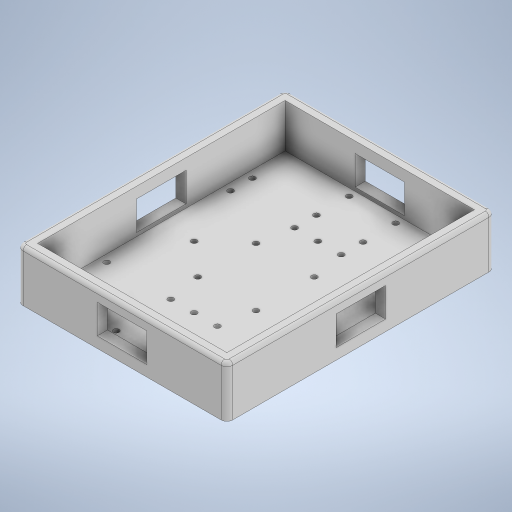
# Autodesk Inventor part: base
Saved by Autodesk Inventor 2024 (Build 280153000, 153)
## iProperties
Created: 2023-11-06
Part Number: base
Material: Generic
Document SubType Name: Modeling
Designer: dimademler
Density: 1 g/cm^3
Appearance: Default
Author: dimademler
Autodesk Inventor part; units mm, degrees
ref_plane "YZ Plane" through (0, 0, 0) normal (1, 0, 0) x (0, 1, 0)
ref_plane "XZ Plane" through (0, 0, 0) normal (0, 1, 0) x (-1, 0, 0)
ref_plane "XY Plane" through (0, 0, 0) normal (0, 0, 1) x (1, 0, 0)
sketch "Sketch2" plane through (0, 0, 0) normal (0, 1, 0) x (-1, 0, 0)
  line L0 (0, 0) -> (177.8, 0)
  line L1 (177.8, 0) -> (177.8, 228.6)
  line L2 (177.8, 228.6) -> (0, 228.6)
  line L3 (0, 228.6) -> (0, 0)
  dimension "d0" = 177.8
  dimension "d1" = 228.6
  constraints: 8 end point, 2 parallel, 1 horizontal, 1 perpendicular
  measures "d0" distance of L2.end L1.end
  measures "d1" distance of L1.end L0.end
extrude "Extrusion1" add sketch "Sketch2" along normal blind 6.35
sketch "Sketch3" plane through (0, 6.35, 0) normal (0, 1, 0) x (1, 0, 0)
  line L0 (-177.8, -228.6) -> (0, -228.6) projected
  line L1 (-177.8, 0) -> (-177.8, -228.6) projected
  line L2 (0, 0) -> (-177.8, 0) projected
  line L3 (0, -228.6) -> (0, 0) projected
  line L4 (-88.9, -228.6) -> (-88.9, -222.25) construction
  line L5 (-88.9, 0) -> (-88.9, -6.35) construction
  line L6 (-177.8, -114.3) -> (-171.45, -114.3) construction
  line L7 (0, -114.3) -> (-6.35, -114.3) construction
  line L8 (-171.45, -114.3) -> (-171.45, -6.35)
  line L9 (-171.45, -114.3) -> (-171.45, -222.25)
  line L10 (-171.45, -6.35) -> (-88.9, -6.35)
  line L11 (-6.35, -6.35) -> (-88.9, -6.35)
  line L12 (-6.35, -6.35) -> (-6.35, -114.3)
  line L13 (-6.35, -114.3) -> (-6.35, -222.25)
  line L14 (-6.35, -222.25) -> (-88.9, -222.25)
  line L15 (-171.45, -222.25) -> (-88.9, -222.25)
  line L16 (-177.8, -228.6) -> (0, -228.6)
  line L17 (0, -228.6) -> (0, 0)
  line L18 (0, 0) -> (-177.8, 0)
  line L19 (-177.8, 0) -> (-177.8, -228.6)
  dimension "d4" = 6.35
  dimension "d5" = 6.35
  dimension "d6" = 6.35
  dimension "d7" = 6.35
  constraints: 32 end point, 5 vertical, 4 equal length, 4 horizontal, 4 midpoint, 2 perpendicular, 2 point on line
  measures "d4" distance of L4.start L4.end
  measures "d5" distance of L5.start L5.end
  measures "d6" distance of L6.start L6.end
  measures "d7" distance of L7.start L7.end
extrude "Extrusion2" add sketch "Sketch3" along normal blind 38.1
sketch "Sketch4" plane through (0, 0, 0) normal (0, -1, 0) x (1, 0, 0)
  line L0 (-177.8, 0) -> (-177.8, 228.6) projected
  line L1 (-177.8, 228.6) -> (0, 228.6) construction
  line L2 (0, 228.6) -> (0, 0) projected
  line L3 (0, 0) -> (-177.8, 0) projected
  line L4 (-88.9, 228.6) -> (-88.9, 0) construction
  line L5 (0, 114.3) -> (-177.8, 114.3) construction
  line L6 (-88.9, 228.6) -> (-68.58, 228.6)
  line L7 (0, 228.6) -> (-177.8, 228.6) construction
  line L8 (-88.9, 228.6) -> (-109.22, 228.6)
  line L9 (-68.58, 228.6) -> (-68.58, 0) construction
  line L10 (-109.22, 228.6) -> (-109.22, 0) construction
  line L11 (-68.58, 228.6) -> (-68.58, 177.8) construction
  line L12 (-109.22, 228.6) -> (-109.22, 177.8) construction
  line L13 (-68.58, 177.8) -> (-68.58, 187.325) construction
  line L14 (-68.58, 177.8) -> (-68.58, 168.275) construction
  circle A0 centre (-68.58, 187.325) radius 2.413
  circle A1 centre (-68.58, 168.275) radius 2.413
  line L15 (-68.58, 187.325) -> (0, 187.325) construction
  line L16 (0, 187.325) -> (-12.7, 187.325) construction
  line L17 (-68.58, 168.275) -> (0, 168.275) construction
  line L18 (0, 168.275) -> (-12.7, 168.275) construction
  circle A2 centre (-12.7, 187.325) radius 2.413
  circle A3 centre (-12.7, 168.275) radius 2.413
  circle A4 centre (-68.58, 215.9) radius 2.413
  circle A5 centre (-109.22, 187.325) radius 2.413
  circle A6 centre (-109.22, 168.275) radius 2.413
  circle A7 centre (-165.1, 187.325) radius 2.413
  circle A8 centre (-165.1, 168.275) radius 2.413
  circle A9 centre (-109.22, 215.9) radius 2.413
  circle A10 centre (-68.58, 41.275) radius 2.413
  circle A11 centre (-68.58, 60.325) radius 2.413
  circle A12 centre (-12.7, 41.275) radius 2.413
  circle A13 centre (-12.7, 60.325) radius 2.413
  circle A14 centre (-68.58, 12.7) radius 2.413
  circle A15 centre (-109.22, 12.7) radius 2.413
  circle A16 centre (-109.22, 41.275) radius 2.413
  circle A17 centre (-165.1, 41.275) radius 2.413
  circle A18 centre (-165.1, 60.325) radius 2.413
  circle A19 centre (-109.22, 60.325) radius 2.413
  dimension "d10" = 20.32
  dimension "d11" = 50.8
  dimension "d12" = 9.525
  dimension "d13" = 4.826
  dimension "d14" = 4.826
  dimension "d16" = 12.7
  dimension "d17" = 4.826
  dimension "d18" = 4.826
  dimension "d19" = 12.7
  dimension "d20" = 4.826
  dimension "d21" = 12.7
  constraints: 30 end point, 20 centre point, 19 symmetric about line, 12 point on line, 4 coincident, 4 midpoint, 2 equal length, 2 perpendicular, 1 parallel, 15 other
  measures "d10" distance of L4.start L6.end
  measures "d11" distance of L6.end L11.end
  measures "d12" distance of L11.end L13.end
  measures "d13" diameter of A0
  measures "d14" diameter of A1
  measures "d16" distance of L15.end L16.end
  measures "d17" diameter of A2
  measures "d18" diameter of A3
  measures "d19" distance of L17.end L18.end
  measures "d20" diameter of A4
  measures "d21" distance from line of L6 A4.centre
extrude "Extrusion3" cut sketch "Sketch4" against normal through all
sketch "Sketch5" plane through (0, 6.35, 0) normal (0, 1, 0) x (1, 0, 0)
  circle A0 centre (-109.22, -187.325) radius 2.413 projected
  circle A1 centre (-68.58, -168.275) radius 2.413 projected
  circle A2 centre (-12.7, -60.325) radius 2.413 projected
  circle A3 centre (-68.58, -12.7) radius 2.413 projected
  circle A4 centre (-165.1, -60.325) radius 2.413 projected
  circle A5 centre (-109.22, -60.325) radius 2.413 projected
  circle A6 centre (-68.58, -60.325) radius 2.413 projected
  circle A7 centre (-12.7, -168.275) radius 2.413 projected
  circle A8 centre (-109.22, -168.275) radius 2.413 projected
  circle A9 centre (-109.22, -215.9) radius 2.413 projected
  circle A10 centre (-165.1, -187.325) radius 2.413 projected
  circle A11 centre (-68.58, -187.325) radius 2.413 projected
  circle A12 centre (-12.7, -41.275) radius 2.413 projected
  circle A13 centre (-109.22, -12.7) radius 2.413 projected
  circle A14 centre (-165.1, -41.275) radius 2.413 projected
  circle A15 centre (-109.22, -41.275) radius 2.413 projected
  circle A16 centre (-68.58, -41.275) radius 2.413 projected
  circle A17 centre (-12.7, -187.325) radius 2.413 projected
  circle A18 centre (-165.1, -168.275) radius 2.413 projected
  circle A19 centre (-68.58, -215.9) radius 2.413 projected
  line L0 (-171.45, -222.25) -> (-6.35, -222.25) projected
  line L1 (-6.35, -222.25) -> (-6.35, -6.35) projected
  line L2 (-6.35, -6.35) -> (-171.45, -6.35) projected
  line L3 (-171.45, -6.35) -> (-171.45, -222.25) projected
  line L4 (-171.45, -114.3) -> (-6.35, -114.3) construction
  line L5 (-88.9, -6.35) -> (-88.9, -222.25) construction
  line L6 (-34.925, -168.275) -> (-142.875, -168.275) construction
  line L7 (-142.875, -168.275) -> (-142.875, -60.325) construction
  line L8 (-142.875, -60.325) -> (-34.925, -60.325) construction
  line L9 (-34.925, -60.325) -> (-34.925, -168.275) construction
  line L10 (-34.925, -168.275) -> (-142.875, -60.325) construction
  line L11 (-142.875, -168.275) -> (-34.925, -60.325) construction
  circle A20 centre (-88.9, -168.275) radius 2.413
  circle A21 centre (-142.875, -114.3) radius 2.413
  circle A22 centre (-88.9, -60.325) radius 2.413
  circle A23 centre (-34.925, -114.3) radius 2.413
  point P0 (0, 0)
  point P1 (-88.9, -114.3)
  dimension "d24" = 107.95
  dimension "d25" = 107.95
  dimension "d26" = 4.826
  dimension "d27" = 4.826
  dimension "d28" = 4.826
  dimension "d29" = 4.826
  constraints: 16 end point, 11 midpoint, 4 centre point, 2 parallel, 1 horizontal, 1 perpendicular
  measures "d24" distance of L7.end L8.end
  measures "d25" distance of L6.end L7.end
  measures "d26" diameter of A20
  measures "d27" diameter of A21
  measures "d28" diameter of A22
  measures "d29" diameter of A23
extrude "Extrusion4" cut sketch "Sketch5" against normal blind 6.35 contours A20 | A21 | A22 | A23
sketch "Sketch8" plane through (0, 6.35, 0) normal (0, 1, 0) x (1, 0, 0)
  circle A0 centre (-88.9, -168.275) radius 2.413 projected
  circle A1 centre (-88.9, -60.325) radius 2.413 projected
  circle A2 centre (-34.925, -114.3) radius 2.413 projected
  circle A3 centre (-142.875, -114.3) radius 2.413 projected
  circle A4 centre (-109.22, -187.325) radius 2.413 projected
  circle A5 centre (-68.58, -168.275) radius 2.413 projected
  circle A6 centre (-12.7, -60.325) radius 2.413 projected
  circle A7 centre (-68.58, -12.7) radius 2.413 projected
  circle A8 centre (-165.1, -60.325) radius 2.413 projected
  circle A9 centre (-109.22, -60.325) radius 2.413 projected
  circle A10 centre (-68.58, -60.325) radius 2.413 projected
  circle A11 centre (-12.7, -168.275) radius 2.413 projected
  circle A12 centre (-109.22, -168.275) radius 2.413 projected
  circle A13 centre (-109.22, -215.9) radius 2.413 projected
  circle A14 centre (-165.1, -187.325) radius 2.413 projected
  circle A15 centre (-68.58, -187.325) radius 2.413 projected
  circle A16 centre (-12.7, -41.275) radius 2.413 projected
  circle A17 centre (-109.22, -12.7) radius 2.413 projected
  circle A18 centre (-165.1, -41.275) radius 2.413 projected
  circle A19 centre (-109.22, -41.275) radius 2.413 projected
  circle A20 centre (-68.58, -41.275) radius 2.413 projected
  circle A21 centre (-12.7, -187.325) radius 2.413 projected
  circle A22 centre (-165.1, -168.275) radius 2.413 projected
  circle A23 centre (-68.58, -215.9) radius 2.413 projected
  line L0 (-171.45, -222.25) -> (-6.35, -222.25) projected
  line L1 (-6.35, -222.25) -> (-6.35, -6.35) projected
  line L2 (-6.35, -6.35) -> (-171.45, -6.35) projected
  line L3 (-171.45, -6.35) -> (-171.45, -222.25) projected
  line L4 (-142.875, -114.3) -> (-34.925, -114.3) construction
  line L5 (-88.9, -60.325) -> (-88.9, -168.275) construction
  line L6 (-114.3, -88.9) -> (-63.5, -88.9) construction
  line L7 (-63.5, -88.9) -> (-63.5, -139.7) construction
  line L8 (-63.5, -139.7) -> (-114.3, -139.7) construction
  line L9 (-114.3, -139.7) -> (-114.3, -88.9) construction
  line L10 (-114.3, -88.9) -> (-63.5, -139.7) construction
  line L11 (-63.5, -88.9) -> (-114.3, -139.7) construction
  circle A24 centre (-114.3, -88.9) radius 2.413
  circle A25 centre (-63.5, -88.9) radius 2.413
  circle A26 centre (-114.3, -139.7) radius 2.413
  circle A27 centre (-63.5, -139.7) radius 2.413
  point P0 (0, 0)
  point P1 (-88.9, -114.3)
  dimension "d38" = 50.8
  dimension "d39" = 50.8
  dimension "d40" = 4.826
  dimension "d41" = 4.826
  dimension "d42" = 4.826
  dimension "d43" = 4.826
  constraints: 16 end point, 4 centre point, 4 coincident, 3 midpoint, 2 horizontal, 2 parallel, 1 perpendicular, 1 vertical
  measures "d38" distance of L7.end L8.end
  measures "d39" distance of L6.end L7.end
  measures "d40" diameter of A24
  measures "d41" diameter of A25
  measures "d42" diameter of A26
  measures "d43" diameter of A27
extrude "Extrusion7" cut sketch "Sketch8" against normal through all contours A24 | A25 | A26 | A27
sketch "Sketch9" plane through (-177.8, 0, 228.6) normal (0, 0, 1) x (1, 0, 0)
  line L0 (177.8, 44.45) -> (0, 44.45) projected
  line L1 (88.9, 44.45) -> (88.9, 0) construction
  line L2 (91.313, 0) -> (86.487, 0) projected
  line L3 (177.8, 0) -> (177.8, 44.45) projected
  line L4 (0, 0) -> (0, 44.45) projected
  line L5 (177.8, 22.225) -> (0, 22.225) construction
  line L6 (67.31, 9.525) -> (110.49, 9.525)
  line L7 (110.49, 9.525) -> (110.49, 34.925)
  line L8 (110.49, 34.925) -> (67.31, 34.925)
  line L9 (67.31, 34.925) -> (67.31, 9.525)
  line L10 (67.31, 9.525) -> (110.49, 34.925) construction
  line L11 (110.49, 9.525) -> (67.31, 34.925) construction
  point P0 (88.9, 22.225)
  dimension "d46" = 43.18
  dimension "d47" = 25.4
  constraints: 16 end point, 7 midpoint, 2 parallel, 1 horizontal, 1 perpendicular
  measures "d46" distance of L7.end L8.end
  measures "d47" distance of L6.end L7.end
extrude "Extrusion8" cut sketch "Sketch9" against normal through all
sketch "Sketch10" plane through (0, 0, 228.6) normal (1, 0, 0) x (0, 0, -1)
  line L0 (0, 0) -> (228.6, 0) projected
  line L1 (228.6, 0) -> (228.6, 44.45) projected
  line L2 (0, 44.45) -> (228.6, 44.45) projected
  line L3 (0, 0) -> (0, 44.45) projected
  line L4 (0, 22.225) -> (228.6, 22.225) construction
  line L5 (114.3, 44.45) -> (114.3, 0) construction
  line L6 (92.71, 9.525) -> (135.89, 9.525)
  line L7 (135.89, 9.525) -> (135.89, 34.925)
  line L8 (135.89, 34.925) -> (92.71, 34.925)
  line L9 (92.71, 34.925) -> (92.71, 9.525)
  line L10 (92.71, 9.525) -> (135.89, 34.925) construction
  line L11 (135.89, 9.525) -> (92.71, 34.925) construction
  point P0 (114.3, 22.225)
  dimension "d50" = 43.18
  dimension "d51" = 25.4
  constraints: 16 end point, 7 midpoint, 2 parallel, 1 horizontal, 1 perpendicular
  measures "d50" distance of L8.end L7.end
  measures "d51" distance of L7.end L6.end
extrude "Extrusion9" cut sketch "Sketch10" against normal through all contours L9 L8 L7 L6
sketch "Sketch11" plane through (-177.8, 0, 228.6) normal (0, 0, 1) x (1, 0, 0)
  line L0 (67.31, 34.925) -> (110.49, 34.925) projected
  line L1 (110.49, 34.925) -> (110.49, 9.525) projected
  line L2 (110.49, 9.525) -> (67.31, 9.525) projected
  line L3 (67.31, 9.525) -> (67.31, 34.925) projected
  line L4 (0, 0) -> (177.8, 0) projected
  line L5 (177.8, 0) -> (177.8, 44.45) projected
  line L6 (0, 44.45) -> (177.8, 44.45) projected
  line L7 (0, 0) -> (0, 44.45) projected
  point P0 (177.8, 0)
extrude "Extrusion10" add sketch "Sketch11" along normal blind 2.54
sketch "Sketch12" plane through (0, 0, 0) normal (1, 0, 0) x (0, 0, -1)
  line L0 (-135.89, 34.925) -> (-92.71, 34.925) projected
  line L1 (-92.71, 34.925) -> (-92.71, 9.525) projected
  line L2 (-92.71, 9.525) -> (-135.89, 9.525) projected
  line L3 (-135.89, 9.525) -> (-135.89, 34.925) projected
  line L4 (0, 0) -> (-231.14, 0) projected
  line L5 (0, 0) -> (0, 44.45) projected
  line L6 (0, 44.45) -> (-231.14, 44.45) projected
  line L7 (-231.14, 0) -> (-231.14, 44.45) projected
  line L8 (0, 34.925) -> (0, 9.525) projected
  line L9 (0, 9.525) -> (0, 34.925) projected
  line L10 (0, 0) -> (0, 44.45) projected
  line L11 (0, 0) -> (0, 44.45) projected
extrude "Extrusion11" add sketch "Sketch12" along normal blind 2.54
sketch "Sketch13" plane through (-177.8, 0, 0) normal (0, 0, -1) x (-1, 0, 0)
  line L0 (-110.49, 34.925) -> (-67.31, 34.925) projected
  line L1 (-67.31, 34.925) -> (-67.31, 9.525) projected
  line L2 (-67.31, 9.525) -> (-110.49, 9.525) projected
  line L3 (-110.49, 9.525) -> (-110.49, 34.925) projected
  line L4 (0, 0) -> (-180.34, 0) projected
  line L5 (0, 0) -> (0, 44.45) projected
  line L6 (0, 44.45) -> (-180.34, 44.45) projected
  line L7 (-180.34, 0) -> (-180.34, 44.45) projected
  point P0 (-177.8, 0)
extrude "Extrusion12" add sketch "Sketch13" along normal blind 2.54
sketch "Sketch14" plane through (-177.8, 0, 231.14) normal (-1, 0, 0) x (0, 0, 1)
  line L0 (-138.43, 34.925) -> (-95.25, 34.925) projected
  line L1 (-95.25, 34.925) -> (-95.25, 9.525) projected
  line L2 (-95.25, 9.525) -> (-138.43, 9.525) projected
  line L3 (-138.43, 9.525) -> (-138.43, 34.925) projected
  line L4 (-233.68, 0) -> (0, 0) projected
  line L5 (0, 44.45) -> (0, 0) projected
  line L6 (0, 44.45) -> (-233.68, 44.45) projected
  line L7 (-233.68, 0) -> (-233.68, 44.45) projected
  point P0 (-231.14, 0)
extrude "Extrusion13" add sketch "Sketch14" along normal blind 2.54
fillet "Fillet1" radius 5.08 1 edges at (-180.34, 22.225, 231.14)
fillet "Fillet2" radius 5.08 1 edges at (2.54, 22.225, -2.54)
fillet "Fillet3" radius 5.08 1 edges at (2.54, 22.225, 231.14)
fillet "Fillet4" radius 5.08 1 edges at (-180.34, 22.225, -2.54)
fillet "Fillet5" radius 3.175 4 edges at (-88.9, 44.45, -2.54) (2.54, 44.45, 114.3) (-88.9, 44.45, 231.14) (-180.34, 44.45, 114.3)
equation "\"d2\" = base_thickness"
equation "\"d4\" = base_thickness"
equation "\"d5\" = base_thickness"
equation "\"d6\" = base_thickness"
equation "\"d7\" = base_thickness"
equation "\"d10\" = motor_adapter_across"
equation "\"d12\" = 0.5 * motor_adapter_width"
equation "\"d19\" = d16"
equation "\"d21\" = d16"
equation "\"base_thickness\" = 6.35"
equation "\"motor_adapter_width\" = 19.05"
equation "\"motor_adapter_across\" = 20.32"
body "Solid1"
